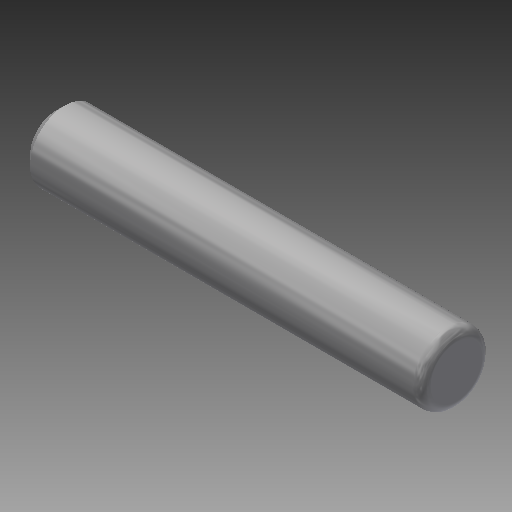
# Autodesk Inventor part: Shaft
Saved by Autodesk Inventor 2017 (Build 210142000, 142)
## iProperties
Created: 2016-12-06
Part Number: Shaft
Material: Steel
Document SubType Name: Modeling
Designer: aesen
Density: 1 g/cm^3
Appearance: Steel
CustomPartVersion: 1
Author: aesen
Autodesk Inventor part; units mm, degrees
ref_plane "Start Plane" through (0, 0, 0) normal (1, 0, 0) x (0, 1, 0)
ref_plane "XZ Plane" through (0, 0, 0) normal (0, 1, 0) x (-1, 0, 0)
ref_plane "XY Plane" through (0, 0, 0) normal (0, 0, 1) x (1, 0, 0)
sketch "Main Sketch" plane through (0, 0, 0) normal (0, 0, 1) x (1, 0, 0)
  line L0 (0, 0) -> (109.7534, 0)
  line L1 (0, 0) -> (0, 9.525)
  line L2 (109.7534, 9.525) -> (109.7534, 0)
  line L3 (0, 9.525) -> (109.7534, 9.525)
  dimension "d3" = 19.05
  constraints: 8 end point, 3 horizontal, 2 vertical
  measures "d3" diameter of L3 L0
revolve "Revolution1" add sketch "Main Sketch" angle 360 about axis through (0, 0, 0) along (1, 0, 0)
chamfer "Chamfer1" distance 2.54 angle 45 1 edges at (0, -9.525, 0) measured on face at (73.1689, 9.4941, -0.7664)
fillet "Fillet1" radius 2.54 1 edges at (109.7534, -9.525, 0)
body "Solid1"
